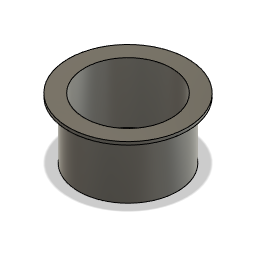
pot v3 (Autodesk Fusion 360 design; units mm, degrees)
Autodesk Fusion 360 part; units mm, degrees
note: some values were not read from the file. Set by a fixed rule: which sketch regions a step uses.
sketch "スケッチ1" plane through (0, 0, 0) normal (0, 1, 0) x (1, 0, 0)
  line L0 (115.8209, 0) -> (-126.022, 0) construction
  line L1 (0, -92.6498) -> (0, 100.0832) construction
  circle A0 centre (0, 0) radius 24.5
  circle A1 centre (0, 0) radius 29.5
  circle A2 centre (0, 0) radius 21.5
  line L2 (21.3542, -2.5) -> (-21.3542, -2.5)
  line L3 (21.3542, 2.5) -> (-21.3542, 2.5)
  line L4 (2.5, -21.3542) -> (2.5, 21.3542)
  line L5 (-2.5, 21.4531) -> (-2.5, -21.3542)
  circle A3 centre (0, 0) radius 12.5
  circle A4 centre (0, 0) radius 15.5
  dimension "d1" = 49
  dimension "d2" = 59
  dimension "d3" = 43
  dimension "d4" = 2.5
  dimension "d5" = 2.5
  dimension "d6" = 2.5
  dimension "d7" = 2.5
  dimension "d8" = 25
  dimension "d9" = 31
  constraint horizontal L0
  constraint perpendicular L0 L1
  constraint coincident A0.centre A1.centre
  constraint concentric A0 A2
  constraint perpendicular L1 L2
  constraint parallel L0 L3
  constraint coincident A2 L2.end
  constraint coincident A2 L3.end
  constraint coincident A2 L2.start
  constraint coincident A2 L3.start
  constraint parallel L1 L4
  constraint parallel L1 L5
  constraint coincident A2 L5.end
  constraint coincident A2 L4.start
  constraint coincident A2 L4.end
  measures "d1" diameter of A0
  measures "d2" diameter of A1
  measures "d3" diameter of A2
  measures "d4" distance of L0 L2
  measures "d5" distance of L0 L3
  measures "d6" distance of L1 L4
  measures "d7" distance of L1 L5
  measures "d8" diameter of A3
  measures "d9" diameter of A4
extrude "押し出し1" add sketch "スケッチ1" along normal blind 2 contours A2 L2 L3 A4 | A2 L4 L5 A4 | L2 L3 A3 A4 | L3 L4 A3 A4 | A2 L4 L5 A4 | L2 L4 A3 A4 | L4 L5 A3 A4 | L2 L3 L4 A3 | L4 L5 A3 A4 | A2 L2 L3 A4 | L3 L5 A3 A4 | L3 L4 L5 A3 | L2 L3 L4 L5 | L2 L5 A3 A4 | L2 L4 L5 A3 | L2 L3 A3 A4 | L2 L3 L5 A3
extrude "押し出し2" add sketch "スケッチ1" along normal blind 30 contours A0
extrude "押し出し3" add sketch "スケッチ1" against normal blind 1.5 from surface at 30 contours A1
